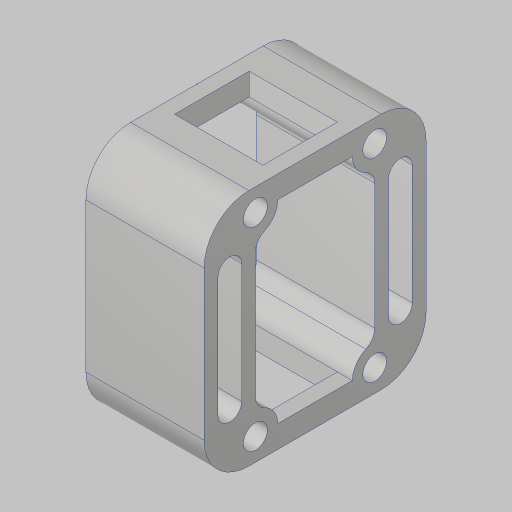
# Autodesk Inventor part: EL2-022
Saved by Autodesk Inventor 2023.5 (Build 275446000, 446)
## iProperties
Created: 2025-02-07
Part Number: EL2-022
Material: Aluminum 6061
Document SubType Name: Modeling
Designer: slick
Density: 2.7 g/cm^3
Appearance: Aluminum - Flat
Author: slick
Autodesk Inventor part; units mm, degrees
ref_plane "YZ Plane" through (0, 0, 0) normal (1, 0, 0) x (0, 1, 0)
ref_plane "XZ Plane" through (0, 0, 0) normal (0, 1, 0) x (-1, 0, 0)
ref_plane "XY Plane" through (0, 0, 0) normal (0, 0, 1) x (1, 0, 0)
sketch "Sketch1" plane through (0, 0, 0) normal (1, 0, 0) x (0, 1, 0)
  line L0 (-20.6375, -12.7) -> (20.6375, -12.7) construction
  line L1 (20.6375, -12.7) -> (20.6375, 12.7) construction
  line L2 (20.6375, 12.7) -> (-20.6375, 12.7) construction
  line L3 (-20.6375, 12.7) -> (-20.6375, -12.7) construction
  line L4 (-20.6375, -12.7) -> (20.6375, 12.7) construction
  line L5 (20.6375, -12.7) -> (-20.6375, 12.7) construction
  circle A0 centre (-20.6375, 12.7) radius 4.7625 construction
  circle A1 centre (-20.6375, -12.7) radius 4.7625 construction
  circle A2 centre (20.6375, -12.7) radius 4.7625 construction
  circle A3 centre (20.6375, 12.7) radius 4.7625 construction
  line L6 (-25.4, -23.622) -> (25.4, -23.622)
  line L7 (25.4, -23.622) -> (25.4, 23.622)
  line L8 (25.4, 23.622) -> (-25.4, 23.622)
  line L9 (-25.4, 23.622) -> (-25.4, -23.622)
  line L10 (-25.4, -23.622) -> (25.4, 23.622) construction
  line L11 (25.4, -23.622) -> (-25.4, 23.622) construction
  line L12 (20.6375, -7.9375) -> (20.6375, 7.9375)
  line L13 (15.875, -12.7) -> (-15.875, -12.7)
  line L14 (-20.6375, 7.9375) -> (-20.6375, -7.9375)
  line L15 (-15.875, 12.7) -> (15.875, 12.7)
  arc A4 (15.875, 12.7) -> (20.6375, 7.9375) centre (20.6375, 12.7) ccw
  arc A5 (20.6375, -7.9375) -> (15.875, -12.7) centre (20.6375, -12.7) ccw
  arc A6 (-15.875, -12.7) -> (-20.6375, -7.9375) centre (-20.6375, -12.7) ccw
  arc A7 (-20.6375, 7.9375) -> (-15.875, 12.7) centre (-20.6375, 12.7) ccw
  line L16 (12.7, 18.161) -> (-12.7, 18.161) construction
  line L17 (12.7, 20.701) -> (-12.7, 20.701)
  line L18 (-12.7, 15.621) -> (12.7, 15.621)
  arc A8 (12.7, 15.621) -> (12.7, 20.701) centre (12.7, 18.161) ccw
  arc A9 (-12.7, 20.701) -> (-12.7, 15.621) centre (-12.7, 18.161) ccw
  line L19 (12.7, -18.161) -> (-12.7, -18.161) construction
  line L20 (12.7, -20.701) -> (-12.7, -20.701)
  line L21 (-12.7, -15.621) -> (12.7, -15.621)
  arc A10 (12.7, -20.701) -> (12.7, -15.621) centre (12.7, -18.161) ccw
  arc A11 (-12.7, -15.621) -> (-12.7, -20.701) centre (-12.7, -18.161) ccw
  line L22 (0, 23.622) -> (0, 12.7) construction
  line L23 (0, -12.7) -> (0, -23.622) construction
  point P0 (0, 0)
  point P1 (0, 18.161)
  point P2 (0, -18.161)
  point P3 (0, 18.161)
  point P4 (0, -18.161)
  dimension "d0" = 25.4
  dimension "d1" = 41.275
  dimension "d2" = 9.525
  dimension "d3" = 47.244
  dimension "d4" = 2.54
  dimension "d5" = 25.4
  constraints: 52 end point, 24 point on circle, 14 coincident, 12 centre point, 12 midpoint, 9 point on line, 9 tangent, 7 parallel, 4 equal radius, 4 vertical alignment, 3 horizontal, 2 perpendicular
  measures "d0" distance of L0.end L1.end
  measures "d1" distance of L1.end L2.end
  measures "d2" diameter of A0
  measures "d3" distance between parallel lines of L6 L8
  measures "d4" radius of A8
  measures "d5" distance of L16.start L16.end
extrude "Extrusion1" add sketch "Sketch1" along normal blind 25.146
hole "Hole1" at (0, 20.6375, 12.7) at (0, 20.6375, -12.7) at (0, -20.6375, -12.7) at (0, -20.6375, 12.7) direction (1, 0, 0) diameter 5.1054 end through all clearance for "Flat Head Machine Screw (82)" size "#10" standard "Ansi Unified Screw Threads"
sketch "Sketch2" plane through (0, 25.4, 23.622) normal (0, 1, 0) x (1, 0, 0)
  point P0 (0, 23.622)
sketch "Sketch3" plane through (0, 25.4, 23.622) normal (0, 1, 0) x (1, 0, 0)
  line L0 (3.175, 15.6845) -> (21.9634, 15.6845)
  line L1 (21.9634, 15.6845) -> (21.9634, 31.5595)
  line L2 (21.9634, 31.5595) -> (3.175, 31.5595)
  line L3 (3.175, 31.5595) -> (3.175, 15.6845)
  line L4 (3.175, 15.6845) -> (21.9634, 31.5595) construction
  line L5 (21.9634, 15.6845) -> (3.175, 31.5595) construction
  line L6 (0, 47.244) -> (0, 0) construction
  line L7 (25.146, 47.244) -> (25.146, 0) construction
  line L8 (0, 15.6845) -> (25.146, 15.6845) construction
  point P0 (0, 23.622)
  point P1 (12.5692, 23.622)
  point P2 (21.9634, 23.622)
  point P3 (3.175, 23.622)
  point P4 (0, 23.622)
  point P5 (0, 23.622)
  point P6 (25.146, 23.622)
  dimension "d16" = 3.175
  dimension "d17" = 3.1826
  constraints: 12 end point, 7 midpoint, 2 horizontal alignment, 2 parallel, 1 horizontal, 1 perpendicular
  measures "d16" distance of point (0, 23.622) point (3.175, 23.622)
  measures "d17" distance from line of point (25.146, 23.622) L1
extrude "Extrusion2" cut sketch "Sketch3" against normal through all
fillet "Fillet1" radius 3.175 4 edges at (12.573, 15.875, 12.7) (12.573, 15.875, -12.7) (12.573, -15.875, -12.7) (12.573, -15.875, 12.7)
fillet "Fillet2" radius 9.525 4 edges at (12.573, -25.4, -23.622) (12.573, -25.4, 23.622) (12.573, 25.4, 23.622) (12.573, 25.4, -23.622)
body "Solid1"
